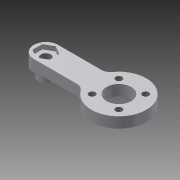
# Autodesk Inventor part: link_short
Saved by Autodesk Inventor 2014 (Build 180170000, 170)
## iProperties
Created: 2015-03-09
Part Number: link_short
Material: 一般
Document SubType Name: Modeling
Designer: Hideyuki Takei
Density: 1 g/cm^3
Appearance: 既定
Author: Hideyuki Takei
Autodesk Inventor part; units mm, degrees
ref_plane "YZ Plane" through (0, 0, 0) normal (1, 0, 0) x (0, 1, 0)
ref_plane "XZ Plane" through (0, 0, 0) normal (0, 1, 0) x (-1, 0, 0)
ref_plane "XY Plane" through (0, 0, 0) normal (0, 0, 1) x (1, 0, 0)
sketch "スケッチ1" plane through (0, 0, 0) normal (0, 0, 1) x (1, 0, 0)
  line L0 (0, 0) -> (24, 0) construction
  arc A0 (0, 4) -> (0, -4) centre (0, 0) ccw
  circle A1 centre (0, 0) radius 1.6
  circle A2 centre (24, 0) radius 4.05
  circle A3 centre (24, 0) radius 9
  circle A4 centre (19.6, 4.4) radius 1.05
  circle A5 centre (28.4, 4.4) radius 1.05
  circle A6 centre (19.6, -4.4) radius 1.05
  circle A7 centre (28.4, -4.4) radius 1.05
  line L1 (0, 4) -> (15.9377, 4)
  line L2 (0, -4) -> (15.9377, -4)
  point P0 (12, 0)
  dimension "d0" = 24
  dimension "d1" = 4
  dimension "d2" = 3.2
  dimension "d3" = 8.1
  dimension "d6" = 18
  dimension "d7" = 8.8
  dimension "d8" = 8.8
  dimension "d9" = 4.4
  dimension "d10" = 4.4
  dimension "d11" = 2.1
  dimension "d12" = 2.1
  dimension "d13" = 2.1
  dimension "d14" = 2.1
  dimension "d15" = 8.8
  dimension "d16" = 8.8
  dimension "d17" = 4.4
  dimension "d18" = 4.4
  constraints: 8 centre point, 8 end point, 4 point on circle, 3 coincident, 2 parallel, 2 tangent, 1 horizontal, 1 midpoint
  measures "d0" distance of L0.start L0.end
  measures "d1" radius of A0
  measures "d2" diameter of A1
  measures "d3" diameter of A2
  measures "d6" diameter of A3
  measures "d7" distance of A5.centre A4.centre
  measures "d8" distance of A7.centre A6.centre
  measures "d9" horizontal distance of A7.centre L0.end
  measures "d10" horizontal distance of L0.end A5.centre
  measures "d11" diameter of A4
  measures "d12" diameter of A5
  measures "d13" diameter of A6
  measures "d14" diameter of A7
  measures "d15" distance of A7.centre A5.centre
  measures "d16" distance of A6.centre A4.centre
  measures "d17" horizontal distance of A5.centre L0.end
  measures "d18" horizontal distance of L0.end A4.centre
extrude "押し出し1" add sketch "スケッチ1" along normal blind 3.5
sketch "スケッチ3" plane through (0, 0, 0) normal (0, 0, 1) x (1, 0, 0)
  circle A0 centre (0, 0) radius 4
  circle A1 centre (0, 0) radius 1.6
  dimension "d20" = 8
  dimension "d21" = 3.2
  constraints: 2 centre point, 2 coincident
  measures "d20" diameter of A0
  measures "d21" diameter of A1
extrude "押し出し2" add sketch "スケッチ3" against normal blind 0.5
sketch "スケッチ4" plane through (0, 0, 0) normal (0, 0, 1) x (1, 0, 0)
  circle A0 centre (0, 0) radius 2.5
  circle A1 centre (0, 0) radius 1.6
  dimension "d24" = 3.2
  dimension "d25" = 5
  constraints: 2 centre point, 2 coincident
  measures "d24" diameter of A1
  measures "d25" diameter of A0
extrude "押し出し3" add sketch "スケッチ4" against normal blind 3.7
sketch "スケッチ5" plane through (0, 0, 3.5) normal (0, 0, 1) x (1, 0, 0)
  circle A0 centre (0, 0) radius 1.6 projected
  arc A1 (0, 4) -> (0, -4) centre (0, 0) ccw projected
  line L0 (0, 3.2332) -> (2.8, 1.6166)
  line L1 (2.8, 1.6166) -> (2.8, -1.6166)
  line L2 (2.8, -1.6166) -> (0, -3.2332)
  line L3 (0, -3.2332) -> (-2.8, -1.6166)
  line L4 (-2.8, -1.6166) -> (-2.8, 1.6166)
  line L5 (-2.8, 1.6166) -> (0, 3.2332)
  dimension "d28" = 5.6
  constraints: 12 end point, 1 coincident, 13 other
  measures "d28" distance between parallel lines of L1 L4
extrude "押し出し4" cut sketch "スケッチ5" against normal blind 1.5
fillet "フィレット1" radius 3 2 edges at (15.9377, -4, 1.75) (15.9377, 4, 1.75)
sketch "スケッチ6" plane through (0, 0, 0) normal (0, 0, 1) x (1, 0, 0)
  line L0 (0, 0) -> (24, 0) construction
  arc A0 (0, 4) -> (0, -4) centre (0, 0) ccw
  circle A1 centre (0, 0) radius 1.6
  circle A2 centre (24, 0) radius 4.05
  circle A3 centre (24, 0) radius 8.5
  circle A4 centre (19.6, 4.4) radius 1.05
  circle A5 centre (28.4, 4.4) radius 1.05
  circle A6 centre (19.6, -4.4) radius 1.05
  circle A7 centre (28.4, -4.4) radius 1.05
  line L1 (0, 4) -> (16.5, 4)
  line L2 (0, -4) -> (16.5, -4)
  line L3 (17.3888, 5.0664) -> (19.0715, 6.6481)
  line L4 (19.0715, 6.6481) -> (21.2827, 5.9817)
  line L5 (21.2827, 5.9817) -> (21.8112, 3.7336)
  line L6 (21.8112, 3.7336) -> (20.1285, 2.1519)
  line L7 (20.1285, 2.1519) -> (17.9173, 2.8183)
  line L8 (17.9173, 2.8183) -> (17.3888, 5.0664)
  line L9 (26.7709, 6.0369) -> (29.0031, 6.6293)
  line L10 (29.0031, 6.6293) -> (30.6321, 4.9923)
  line L11 (30.6321, 4.9923) -> (30.0291, 2.7631)
  line L12 (30.0291, 2.7631) -> (27.7969, 2.1707)
  line L13 (27.7969, 2.1707) -> (26.1679, 3.8077)
  line L14 (26.1679, 3.8077) -> (26.7709, 6.0369)
  line L15 (17.9287, -2.8062) -> (20.1446, -2.1557)
  line L16 (20.1446, -2.1557) -> (21.8159, -3.7495)
  line L17 (21.8159, -3.7495) -> (21.2713, -5.9938)
  line L18 (21.2713, -5.9938) -> (19.0554, -6.6443)
  line L19 (19.0554, -6.6443) -> (17.3841, -5.0505)
  line L20 (17.3841, -5.0505) -> (17.9287, -2.8062)
  line L21 (29.0633, -6.6121) -> (26.8159, -6.0805)
  line L22 (26.8159, -6.0805) -> (26.1526, -3.8684)
  line L23 (26.1526, -3.8684) -> (27.7367, -2.1879)
  line L24 (27.7367, -2.1879) -> (29.9841, -2.7195)
  line L25 (29.9841, -2.7195) -> (30.6474, -4.9316)
  line L26 (30.6474, -4.9316) -> (29.0633, -6.6121)
  point P0 (12, 0)
  dimension "d32" = 24
  dimension "d33" = 4
  dimension "d34" = 3.2
  dimension "d35" = 8.1
  dimension "d36" = 17
  dimension "d37" = 8.8
  dimension "d38" = 8.8
  dimension "d39" = 4.4
  dimension "d40" = 4.4
  dimension "d41" = 2.1
  dimension "d42" = 2.1
  dimension "d43" = 2.1
  dimension "d44" = 2.1
  dimension "d45" = 8.8
  dimension "d46" = 8.8
  dimension "d47" = 4.4
  dimension "d48" = 4.4
  dimension "d49" = 4
  dimension "d50" = 4
  dimension "d51" = 4
  dimension "d52" = 4
  constraints: 56 end point, 8 centre point, 7 coincident, 4 point on circle, 2 parallel, 2 tangent, 1 horizontal, 1 midpoint, 52 other
  measures "d32" distance of L0.start L0.end
  measures "d33" radius of A0
  measures "d34" diameter of A1
  measures "d35" diameter of A2
  measures "d36" diameter of A3
  measures "d37" distance of A5.centre A4.centre
  measures "d38" distance of A7.centre A6.centre
  measures "d39" horizontal distance of A7.centre L0.end
  measures "d40" horizontal distance of L0.end A5.centre
  measures "d41" diameter of A4
  measures "d42" diameter of A5
  measures "d43" diameter of A6
  measures "d44" diameter of A7
  measures "d45" distance of A7.centre A5.centre
  measures "d46" distance of A6.centre A4.centre
  measures "d47" horizontal distance of A5.centre L0.end
  measures "d48" horizontal distance of L0.end A4.centre
  measures "d49" distance between parallel lines of L7 L4
  measures "d50" distance between parallel lines of L12 L9
  measures "d51" distance between parallel lines of L21 L24
  measures "d52" distance between parallel lines of L18 L15
extrude "押し出し5" cut sketch "スケッチ6" along normal blind 2 contours L3 L4 L5 L6 L7 L8 | L9 L10 L11 L12 L13 L14 | L15 L16 L17 L18 L19 L20 | L21 L22 L23 L24 L25 L26
equation "\"d8\" = d7"
equation "\"d9\" = 0.5 * d8"
equation "\"d10\" = 0.5 * d7"
equation "\"d12\" = d11"
equation "\"d13\" = d11"
equation "\"d14\" = d11"
equation "\"d15\" = d7"
equation "\"d16\" = d7"
equation "\"d17\" = 0.5 * d7"
equation "\"d18\" = 0.5 * d15"
equation "\"d38\" = d37"
equation "\"d39\" = 0.5 * d38"
equation "\"d40\" = 0.5 * d37"
equation "\"d42\" = d41"
equation "\"d43\" = d41"
equation "\"d44\" = d41"
equation "\"d45\" = d37"
equation "\"d46\" = d37"
equation "\"d47\" = 0.5 * d37"
equation "\"d48\" = 0.5 * d45"
